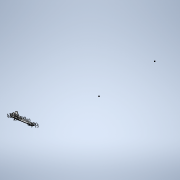
# Autodesk Inventor part: LegEnd_Left_v1
Saved by Autodesk Inventor 2020.3 (Build 243373000, 373)
## iProperties
Created: 2021-02-18
Part Number: LegEnd_Left_v1
Material: Generic
Document SubType Name: Modeling
Designer: sanyi
Density: 1 g/cm^3
Appearance: Default
Author: sanyi
Autodesk Inventor part; units mm, degrees
ref_plane "YZ Plane" through (0, 0, 0) normal (1, 0, 0) x (0, 1, 0)
ref_plane "XZ Plane" through (0, 0, 0) normal (0, 1, 0) x (-1, 0, 0)
ref_plane "XY Plane" through (0, 0, 0) normal (0, 0, 1) x (1, 0, 0)
sketch "Sketch1" plane through (0, 0, 0) normal (0, 1, 0) x (-1, 0, 0)
  line L0 (0, 0) -> (-4, 0)
  line L1 (0, 0) -> (0, 35)
  line L2 (-22.2, 0) -> (-22.2, 35)
  line L3 (-17.2, 6) -> (-5, 6)
  line L4 (-5, 6) -> (-5, 29)
  line L5 (-5, 29) -> (-17.2, 29)
  line L6 (-17.2, 29) -> (-17.2, 6)
  line L7 (-22.2, 35) -> (-18.2, 35) construction
  arc A0 (-15.1221, 111.5021) -> (-18.4851, 115.3231) centre (-15, 115) ccw
  arc A1 (-18.4851, 115.3231) -> (-22.2, 35) centre (848.0149, 35) ccw
  line L8 (-11.1, 3.3) -> (-11.1, 31.7) construction
  line L9 (-26.8761, 3.3) -> (8.0494, 3.3) construction
  line L10 (-27.316, 31.7) -> (4.8344, 31.7) construction
  line L11 (-25.0824, 17.5) -> (3.9206, 17.5) construction
  arc A2 (-11.5003, 114.9512) -> (-5, 35) centre (410.9362, 109.0571) ccw
  arc A3 (-16.1214, 94.9732) -> (-18.2, 35) centre (848.0149, 35) ccw
  arc A4 (-15.3097, 95) -> (-9.0623, 35) centre (410.9362, 109.0571) ccw
  line L12 (-18.2, 35) -> (-9.0623, 35)
  line L13 (-5, 35) -> (0, 35)
  line L14 (-16.1214, 94.9732) -> (-15.3097, 95)
  line L15 (-15.3097, 95) -> (-11.3119, 95.1318) construction
  line L16 (-16.1214, 94.9732) -> (-20.1118, 95.2502) construction
  line L17 (-9.0623, 35) -> (-5.1231, 35.6946) construction
  line L18 (-15, 115) -> (-11.5, 115) construction
  line L19 (-15, 115) -> (-15.5584, 99.0097) construction
  line L20 (-17.2, 6) -> (-22.2, 6)
  line L21 (-17.2, 17.5) -> (-22.2, 17.5)
  line L22 (-5, 6) -> (0, 6)
  line L23 (-5, 17.5) -> (0, 17.5)
  arc A5 (-15.2, 0) -> (-14.0457, -5.4507) centre (-1.7538, 0) ccw
  arc A6 (-9.6573, 0) -> (-14.0457, -5.4507) centre (-0.4309, -11.92) ccw
  arc A7 (-18.2, 0) -> (-13, -12) centre (-1.7538, 0) ccw
  arc A8 (-4, 0) -> (-13, -12) centre (1.9602, -13.8452) ccw
  line L24 (-14.0457, -5.4507) -> (-16.7881, -6.6669) construction
  line L25 (-14.0457, -5.4507) -> (-11.3889, -6.8441) construction
  line L26 (-18.2, 0) -> (-22.2, 0)
  line L27 (-15.2, 0) -> (-18.2, 0) construction
  line L28 (-9.6573, 0) -> (-15.2, 0)
  line L29 (-7.7289, -2.2981) -> (-9.6573, 0) construction
  arc A9 (-18.4851, 115.3231) -> (-15.1221, 111.5021) centre (-15, 115) ccw
  line L30 (-19.7, -2.9834) -> (-19.7, 47.0125) construction
  point P0 (-15.2094, 109.0037)
  dimension "d4" = 6
  dimension "d5" = 23
  dimension "d6" = 12.2
  dimension "d7" = 5
  dimension "d15" = 7
  dimension "d17" = 5
  dimension "d18" = 4
  dimension "d21" = 20
  dimension "d23" = 80
  dimension "d24" = 15
  dimension "d29" = 170
  dimension "d30" = 6
  dimension "d31" = 10
  dimension "d43" = 4
  dimension "d44" = 3
  dimension "d45" = 4
  dimension "d50" = 13
  dimension "d51" = 12
  dimension "d52" = 130
  dimension "d53" = 92
  dimension "d95" = 2.7
  constraints: 62 end point, 28 point on circle, 14 point on line, 10 centre point, 9 horizontal, 9 line through centre, 6 equal length, 5 perpendicular, 4 midpoint, 4 vertical, 3 tangent, 2 parallel, 1 collinear, 1 equal radius, 11 other
  measures "d4" distance between parallel lines of L0 L3
  measures "d5" distance between parallel lines of L5 L3
  measures "d6" distance between parallel lines of L4 L6
  measures "d7" distance between parallel lines of L1 L4
  measures "d15" diameter of A0
  measures "d17" distance of L1.end L13.start
  measures "d18" distance of L2.end L7.end
  measures "d21" vertical distance of L18.start L14.end
  measures "d23" vertical distance of L18.start L1.end
  measures "d24" horizontal distance of L1.end L18.start
  measures "d29" angle of L12 L17
  measures "d30" distance of L18.start point (-15.209, 109.004)
  measures "d31" distance of L19.end point (-15.209, 109.004)
  measures "d43" distance of L2.start L26.start
  measures "d44" distance of L27.start L26.start
  measures "d45" distance of L0.start L0.end
  measures "d50" distance from line of L1 A7.end
  measures "d51" distance from line of L26 A7.end
  measures "d52" angle of L28 L29
  measures "d53" angle of L18 L19
  measures "d95" distance between parallel lines of L10 L5
extrude "Extrusion1" add sketch "Sketch1" against normal blind 6 contours L0 A8 A7 L26 L2 L20 L3 L22 L1 | L23 L4 L5 L6 L21 L2 A1 A9 A0 A2 L13 L1 | A0 A9
chamfer "Chamfer1" distance 2.5 angle 45 1 edges at (0, -3, 35)
fillet "Fillet1" radius 3 1 edges at (22.2, -3, 0)
fillet "Fillet1" radius 3 1 edges at (0, -3, 0)
full round fillet "Fillet2" first side at (17.5583, -4, 68.3369) centre faces at (15.8508, -2, 94.9822) second side at (15.0359, -2, 88.2974)
fillet "Fillet3" radius 2 3 edges at (18.2, -3, 35) (9.0623, -3, 35) (5, -3, 35)
fillet "Fillet4" radius 0.5 1 edges at (13, -3, -12)
hole "Hole3" at (11.1, 0, 31.7) at (11.1, 0, 3.3) direction (0, -1, 0) diameter 2.2 end through all
hole "Hole4" at (15.2094, 0, 109.0037) at (15.5584, 0, 99.0097) direction (0, -1, 0) diameter 2.2 end through all
extrude "Extrusion3" add sketch "Sketch1" against normal blind 20.92 contours L22 L4 L23 L1 | L20 L2 L21 L6
fillet "Fillet6" radius 2 4 edges at (0, -13.46, 6) (0, -13.46, 17.5) (22.2, -13.46, 6) (22.2, -13.46, 17.5)
sketch "Sketch2" plane through (0, -20.92, 0) normal (0, -1, 0) x (1, 0, 0)
  line L0 (0, 15.5) -> (0, 8) projected
  line L1 (22.2, 8) -> (22.2, 15.5) projected
  line L2 (11.1, 3.3) -> (11.1, 31.7) construction
  line L3 (19.7, -2.9834) -> (19.7, 47.0125) construction
  line L4 (-2.1013, 11.75) -> (26.032, 11.75) construction
  line L5 (2.5, 8.75) -> (2.5, 14.75) construction
  line L6 (19.7, 8.75) -> (19.7, 14.75) construction
  line L7 (2.5, 8.75) -> (19.7, 8.75) construction
  line L8 (2.5, 14.75) -> (19.7, 14.75) construction
  point P0 (0, 0)
  point P1 (0, 11.75)
  point P2 (22.2, 11.75)
  dimension "d87" = 6
  constraints: 10 end point, 4 coincident, 2 midpoint, 2 perpendicular, 2 point on line, 1 collinear, 1 horizontal, 1 symmetric about line, 1 other
  measures "d87" distance of L5.start L5.end
hole "Hole5" at (2.5, -20.92, 8.75) at (2.5, -20.92, 14.75) at (19.7, -20.92, 8.75) at (19.7, -20.92, 14.75) direction (0, 1, 0) diameter 2 depth 5 tip angle 118
body "Solid1"
